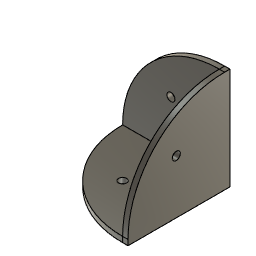
crateCorner v1 (Autodesk Fusion 360 design; units mm, degrees)
Autodesk Fusion 360 part; units mm, degrees
note: some values were not read from the file. Set by a fixed rule: which sketch regions a step uses.
sketch "Sketch3" plane through (0, 0, 0) normal (0, 0, 1) x (1, 0, 0)
  line L0 (10, 15) -> (46, 15)
  line L1 (46, 15) -> (46, 51)
  line L2 (46, 51) -> (10, 51)
  line L3 (10, 51) -> (10, 15)
  line L4 (8, 53) -> (8, 13)
  line L5 (8, 13) -> (48, 13)
  line L6 (48, 13) -> (48, 53)
  line L7 (48, 53) -> (8, 53)
  line L8 (10, 51) -> (10, 53)
  line L9 (10, 51) -> (8, 51)
  line L10 (46, 51) -> (46, 53)
  line L11 (46, 51) -> (48, 51)
  line L12 (46, 15) -> (48, 15)
  line L13 (46, 15) -> (46, 13)
  line L14 (10, 15) -> (10, 13)
  line L15 (10, 15) -> (8, 15)
  dimension "d6" = 36
  dimension "d7" = 36
  dimension "d8" = 2
  constraint horizontal L0
  constraint vertical L1
  constraint horizontal L2
  constraint vertical L3
  constraint coincident L7 L8.end
  constraint perpendicular L7 L8
  constraint coincident L4 L9.end
  constraint perpendicular L4 L9
  constraint coincident L7 L10.end
  constraint perpendicular L7 L10
  constraint coincident L6 L11.end
  constraint perpendicular L6 L11
  constraint coincident L6 L12.end
  constraint perpendicular L6 L12
  constraint perpendicular L0 L13
  constraint coincident L5 L14.end
  constraint perpendicular L5 L14
  constraint coincident L4 L15.end
  constraint perpendicular L4 L15
  measures "d6" distance of L0.start L0.end
  measures "d7" distance of L0.start L2.end
extrude "Extrude1" add sketch "Sketch3" along normal blind 38 contours L1 L6 L11 L12 | L2 L7 L8 L10 | L6 L7 L10 L11
extrude "Extrude2" add sketch "Sketch3" along normal blind 2 contours L0 L1 L2 L3
sketch "Sketch4" plane through (0, 0, 2) normal (0, 0, 1) x (-1, 0, 0)
  line L0 (-10, -51) -> (-10, -15)
  line L1 (-10, -15) -> (-46, -15)
  line L2 (-46, -15) -> (-46, -51)
  line L3 (-46, -51) -> (-10, -51)
  line L4 (-10, -51) -> (-46, -15)
  line L5 (-10, -15) -> (-46, -51)
  circle A0 centre (-28, -33) radius 1.5
  dimension "d13" = 3
  constraint coincident L0.start L3.end
  constraint coincident L1.end L2.start
  constraint coincident L0.end L1.start
  constraint coincident L2.end L3.start
  constraint midpoint L5 A0.centre
  measures "d13" diameter of A0
sketch "Sketch5" plane through (0, 51, 0) normal (0, -1, 0) x (1, 0, 0)
  line L0 (10, 2) -> (46, 2)
  line L1 (46, 2) -> (46, 38)
  line L2 (46, 38) -> (10, 38)
  line L3 (10, 38) -> (10, 2)
  line L4 (10, 38) -> (46, 2)
  line L5 (10, 2) -> (46, 38)
  circle A0 centre (28, 20) radius 1.5
  dimension "d14" = 3
  constraint coincident L2.end L3.start
  constraint coincident L0.end L1.start
  constraint coincident L0.start L3.end
  constraint coincident L1.end L2.start
  constraint midpoint L5 A0.centre
  measures "d14" diameter of A0
sketch "Sketch6" plane through (46, 0, 0) normal (-1, 0, 0) x (0, -1, 0)
  line L0 (-51, 2) -> (-15, 2)
  line L1 (-15, 2) -> (-15, 38)
  line L2 (-15, 38) -> (-51, 38)
  line L3 (-51, 38) -> (-51, 2)
  line L4 (-51, 38) -> (-15, 2)
  line L5 (-51, 2) -> (-15, 38)
  circle A0 centre (-33, 20) radius 1.5
  dimension "d15" = 3
  constraint coincident L2.end L3.start
  constraint coincident L0.end L1.start
  constraint coincident L0.start L3.end
  constraint coincident L1.end L2.start
  constraint midpoint L4 A0.centre
  measures "d15" diameter of A0
extrude "Extrude3" cut sketch "Sketch5" against normal blind 7 contours L4 L5 A0 | L4 L5 A0 | L4 L5 A0 | L4 L5 A0
extrude "Extrude4" cut sketch "Sketch6" against normal blind 10 contours L4 L5 A0 | L4 L5 A0 | L4 L5 A0 | L4 L5 A0
extrude "Extrude5" cut sketch "Sketch4" against normal blind 9 contours L4 L5 A0 | L4 L5 A0 | L4 L5 A0 | L4 L5 A0
fillet "Fillet1" radius 36 3 edges at (10, 52, 38) (10, 15, 1) (47, 15, 38)
